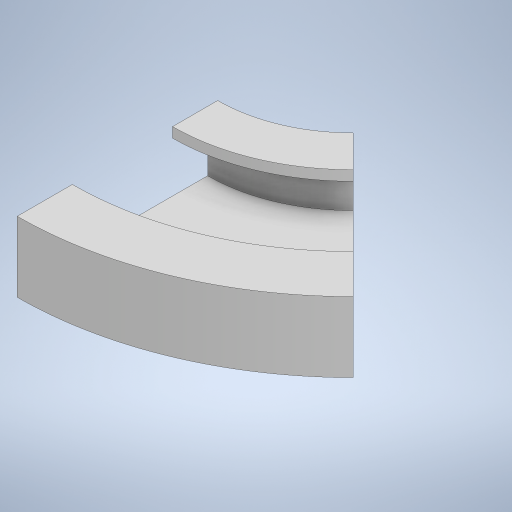
# Autodesk Inventor part: Carousel Fixed Track
Saved by Autodesk Inventor 2023 (Build 270158000, 158)
## iProperties
Created: 2022-11-03
Part Number: Carousel Fixed Track
Material: Generic
Document SubType Name: Modeling
Designer: cheng
Density: 1 g/cm^3
Appearance: Default
Author: cheng
Autodesk Inventor part; units mm, degrees
ref_plane "YZ Plane" through (0, 0, 0) normal (1, 0, 0) x (0, 1, 0)
ref_plane "XZ Plane" through (0, 0, 0) normal (0, 1, 0) x (-1, 0, 0)
ref_plane "XY Plane" through (0, 0, 0) normal (0, 0, 1) x (1, 0, 0)
sketch "Sketch1" plane through (0, 0, 0) normal (0, 1, 0) x (-1, 0, 0)
  circle A0 centre (0, 0) radius 335
  line L0 (335, 0) -> (-335, 0)
  line L1 (0, -335) -> (0, 335)
  line L2 (0, 0) -> (-236.8808, 236.8808)
  line L3 (0, 0) -> (236.8808, -236.8808)
  line L4 (0, 0) -> (236.8808, 236.8808)
  line L5 (0, 0) -> (-236.8808, -236.8808)
  circle A1 centre (0, 0) radius 135
  point P0 (-95.4594, 95.4594)
  point P1 (0, 135)
  dimension "d0" = 670
  dimension "d1" = 45
  dimension "d2" = 45
  dimension "d17" = 200
  constraints: 12 end point, 2 coincident, 2 collinear, 1 centre point, 1 horizontal, 10 other
  measures "d1" angle of L1 L3
  measures "d2" angle of L5 L1
extrude "Extrusion1" add sketch "Sketch1" along normal blind 70 contours L1 A1 L2 A0
sketch "Sketch2" plane through (95.4594, 0, 95.4594) normal (0.7071068, 0, -0.7071068) x (-0.7071068, 0, -0.7071068)
  line L0 (-190, 60) -> (-10, 60)
  line L1 (-10, 60) -> (-10, 10)
  line L2 (-10, 10) -> (-190, 10)
  line L3 (-190, 10) -> (-190, 60)
  line L4 (-200, 0) -> (0, 0) projected
  line L5 (-200, 70) -> (0, 70) projected
  line L6 (-200, 0) -> (-200, 70) projected
  line L7 (0, 0) -> (0, 70) projected
  point P0 (135, 0)
  point P1 (0, 35)
  dimension "d6" = 10
  dimension "d7" = 10
  dimension "d8" = 10
  dimension "d9" = 10
  constraints: 8 end point, 2 parallel, 1 horizontal, 1 midpoint, 1 perpendicular
  measures "d6" distance between parallel lines of L4 L2
  measures "d7" distance between parallel lines of L5 L0
  measures "d8" distance between parallel lines of L6 L3
  measures "d9" distance from line of point (0, 35) L1
sketch3d "3D Sketch1"
  arc A0 (95.4594, 70, 95.4594) -> (0, 70, 135) centre (0, 70, 0) ccw
sweep "Sweep1" cut profiles "Sketch2" path "3D Sketch1" contours L0 L1 L2 L3
sketch "Sketch3" plane through (95.4594, 0, 95.4594) normal (0.7071068, 0, -0.7071068) x (-0.7071068, 0, -0.7071068)
  line L0 (-101.8808, 70) -> (-200, 70) projected
  line L1 (32.4695, 60) -> (-94.8097, 60) projected
  line L2 (-145, 70) -> (-45, 70)
  line L3 (-45, 70) -> (-45, 60)
  line L4 (-45, 60) -> (-145, 60)
  line L5 (-145, 60) -> (-145, 70)
  line L6 (-200, 0) -> (-200, 70) projected
  line L7 (0, 0) -> (0, 70) projected
  point P0 (135, 0)
  dimension "d16" = 100
  dimension "d18" = 45
  constraints: 8 end point, 2 parallel, 2 point on line, 1 horizontal, 1 perpendicular
  measures "d16" distance of L2.start L2.end
  measures "d18" distance between parallel lines of L7 L3
sketch3d "3D Sketch2"
  arc A0 (95.4594, 70, 95.4594) -> (0, 70, 135) centre (0, 70, 0) ccw
sweep "Sweep2" cut profiles "Sketch3" path "3D Sketch2"
body "Solid1"
